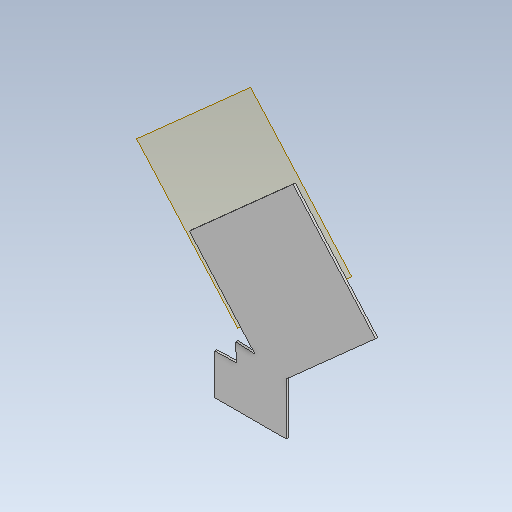
# Autodesk Inventor part: base_plate
Saved by Autodesk Inventor 2020 (Build 240168000, 168)
## iProperties
Created: 2019-07-16
Part Number: base_plate
Material: Générique
Document SubType Name: Modeling
Designer: Thibault
Density: 1 g/cm^3
Appearance: Par défaut
Author: Thibault
Autodesk Inventor part; units mm, degrees
ref_plane "YZ Plane" through (0, 0, 0) normal (1, 0, 0) x (0, 1, 0)
ref_plane "XZ Plane" through (0, 0, 0) normal (0, 1, 0) x (-1, 0, 0)
ref_plane "XY Plane" through (0, 0, 0) normal (0, 0, 1) x (1, 0, 0)
sketch "Anchor (screw side)" plane through (0, 0, 0) normal (0, 0, 1) x (1, 0, 0)
  circle A0 centre (93.7814, 50.2592) radius 0.85
  line L0 (91.2814, 51.2592) -> (88.2814, 51.2592)
  line L1 (88.2814, 51.2592) -> (88.2814, 49.2592)
  line L2 (88.2814, 49.2592) -> (91.2814, 49.2592)
  line L3 (91.2814, 49.2592) -> (91.2814, 51.2592)
  line L4 (99.2814, 51.2592) -> (96.2814, 51.2592)
  line L5 (96.2814, 51.2592) -> (96.2814, 49.2592)
  line L6 (96.2814, 49.2592) -> (99.2814, 49.2592)
  line L7 (99.2814, 49.2592) -> (99.2814, 51.2592)
  line L8 (91.2814, 51.2592) -> (96.2814, 49.2592) construction
  line L9 (96.2814, 51.2592) -> (91.2814, 49.2592) construction
  line L10 (86.6814, 52.8592) -> (100.8814, 52.8592) construction
  line L11 (100.8814, 52.8592) -> (100.8814, 47.6592) construction
  line L12 (100.8814, 47.6592) -> (86.6814, 47.6592) construction
  line L13 (86.6814, 47.6592) -> (86.6814, 52.8592) construction
  point P0 (103.5798, 50.1132)
  dimension "d27" = 1.7
  dimension "d28" = 3
  dimension "d29" = 2
  dimension "d30" = 3
  dimension "d32" = 5
  dimension "d34" = 1.6
  dimension "d35" = 1.6
  dimension "d36" = 1.6
  dimension "d37" = 1.6
  measures "d27" diameter of A0
  measures "d28" distance of L2.end L1.end
  measures "d29" distance of L1.end L0.end
  measures "d30" distance of L6.end L5.end
  measures "d32" distance between parallel lines of L5 L3
  measures "d34" distance between parallel lines of L0 L10
  measures "d35" distance between parallel lines of L12 L2
  measures "d36" distance between parallel lines of L11 L7
  measures "d37" distance between parallel lines of L13 L1
sketch "Anchor (nut side)" plane through (0, 0, 0) normal (0, 0, 1) x (1, 0, 0)
  line L0 (10, 0) -> (8.35, 0)
  line L1 (8.35, 0) -> (8.35, -2.5)
  line L2 (8.35, -2.5) -> (9.15, -2.5)
  line L3 (9.15, -2.5) -> (9.15, -4.5)
  line L4 (5.85, -4.5) -> (5.85, -2.5)
  line L5 (5.85, -2.5) -> (6.65, -2.5)
  line L6 (6.65, -2.5) -> (6.65, 0)
  line L7 (6.65, 0) -> (5, 0)
  line L8 (2, 0) -> (2, 1.75)
  line L9 (2, 0) -> (3, 0) construction
  line L10 (2.25, 2) -> (4.75, 2)
  line L11 (5, 1.75) -> (5, 0)
  line L12 (5, 2) -> (7, 2) construction
  line L13 (10, 0) -> (10, 1.75)
  line L14 (10.25, 2) -> (12.75, 2)
  line L15 (13, 1.75) -> (13, 0)
  line L16 (0, 0) -> (2, 0)
  line L17 (13, 0) -> (15, 0)
  line L18 (5.85, -4.5) -> (6.65, -4.5)
  line L19 (9.15, -4.5) -> (8.35, -4.5)
  line L20 (6.65, -4.5) -> (6.65, -6)
  line L21 (8.35, -4.5) -> (8.35, -6)
  arc A0 (2.25, 2) -> (2, 1.75) centre (2.25, 1.75) ccw
  arc A1 (5, 1.75) -> (4.75, 2) centre (4.75, 1.75) ccw
  arc A2 (10.25, 2) -> (10, 1.75) centre (10.25, 1.75) ccw
  arc A3 (13, 1.75) -> (12.75, 2) centre (12.75, 1.75) ccw
  line L22 (7.15, -6.5) -> (7.85, -6.5)
  arc A4 (6.65, -6) -> (7.15, -6.5) centre (7.15, -6) ccw
  arc A5 (7.85, -6.5) -> (8.35, -6) centre (7.85, -6) ccw
  point P0 (9.1321, -0.6227)
  point P1 (2, 2)
  point P2 (10, 2)
  point P3 (13, 2)
  point P4 (6.65, -6.5)
  point P5 (8.35, -6.5)
  dimension "d3" = 2
  dimension "d5" = 3
  dimension "d7" = 5
  dimension "d8" = 3
  dimension "d10" = 1.65
  dimension "d11" = 2.5
  dimension "d12" = 0.8
  dimension "d13" = 2
  dimension "d14" = 0.8
  dimension "d15" = 1.7
  dimension "d16" = 2.5
  dimension "d18" = 2
  dimension "d19" = 0.8
  dimension "d20" = 0.8
  dimension "d21" = 2
  dimension "d22" = 2
  dimension "d23" = 1.7
  dimension "d24" = 2
  dimension "d25" = 0.25
  dimension "d38" = 2
  dimension "d39" = 0.5
  measures "d3" distance of L16.start L8.start
  measures "d5" distance of point (2, 2) L12.start
  measures "d7" distance of L7.end L0.start
  measures "d8" distance of point (10, 2) point (13, 2)
  measures "d10" distance of L0.start L0.end
  measures "d11" distance of L0.end L1.end
  measures "d12" distance of L1.end L2.end
  measures "d13" distance of L2.end L3.end
  measures "d14" distance of L4.end L5.end
  measures "d15" distance of L6.end L0.end
  measures "d16" distance of L5.end L6.end
  measures "d18" distance of L15.end L17.end
  measures "d19" distance of L4.start L18.end
  measures "d20" distance of L3.end L19.end
  measures "d21" distance of L18.end point (6.65, -6.5)
  measures "d22" distance of L19.end point (8.35, -6.5)
  measures "d23" distance of L18.end L19.end
  measures "d24" distance of L4.start L4.end
  measures "d25" radius of A0
  measures "d38" distance between parallel lines of L16 L10
  measures "d39" radius of A4
ref_plane "Plan de construction1" through (57.5253, 159.7091, 0) normal (0, 0, 1) x (-0.7464987, -0.6653869, 0)
sketch "Esquisse1" plane through (57.5253, 159.7091, 0) normal (0, 0, 1) x (-0.7464987, -0.6653869, 0)
  line L0 (0, 110) -> (103.4714, 110) projected
  line L1 (123.2302, 87.5455) -> (123.2302, 2) projected
  line L2 (0, 0) -> (123.2302, 0) projected
  line L3 (0, 108) -> (0, 2) projected
  line L4 (145.5645, 87.6898) -> (135.4086, 75.5685) projected
  line L5 (108.3469, 112.5474) -> (136.7354, 144.3966) projected
  line L6 (171.4687, 87.8985) -> (170.1379, 86.4055) projected
  line L7 (158.1609, 72.9685) -> (156.8301, 71.4755) projected
  line L8 (108.3469, 112.5474) -> (106.0762, 110)
  line L9 (103.4714, 110) -> (106.0762, 110)
  line L10 (136.7354, 144.3966) -> (184.1541, 102.1302)
  line L11 (184.1541, 102.1302) -> (160.2874, 75.3542)
  line L12 (135.4086, 75.5685) -> (123.2302, 87.5455)
  line L13 (145.5645, 87.6898) -> (160.2874, 75.3542)
  line L14 (123.2302, 2) -> (123.2302, 0)
  line L15 (0, 2) -> (0, 0)
  line L16 (0, 108) -> (0, 110)
  point P0 (149.2109, 80.9461)
  point P1 (170.1379, 86.4055)
  point P2 (171.4687, 87.8985)
  constraints: 18 end point, 4 perpendicular, 3 collinear, 2 equal length
derived "shared_parameters.ipt"
extrude "Extrusion1" add sketch "Esquisse1" along normal blind 2
equation "\"d1\" = sheet_thickness"
equation "\"sheet_thickness\" = 2"
